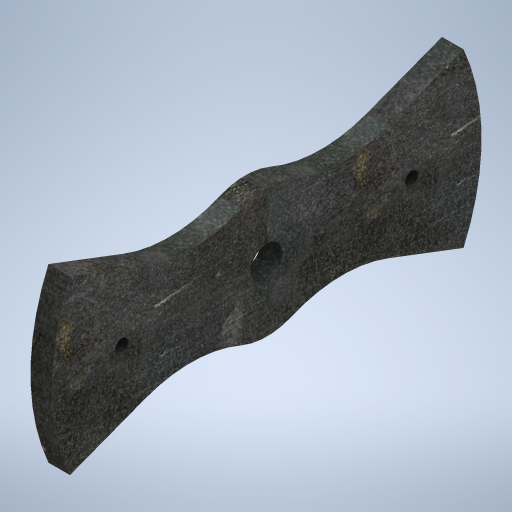
# Autodesk Inventor part: Test weapon
Saved by Autodesk Inventor 2023 (Build 270158000, 158)
## iProperties
Created: 2023-01-06
Part Number: Test weapon
Material: Steel
Document SubType Name: Modeling
Designer: justi
Density: 7.85 g/cm^3
Appearance: Plate
Mass: 1776.63 g
Surface Area: 458.545 cm^2
Volume: 226.322 cm^3
Author: justi
Autodesk Inventor part; units mm, degrees
ref_plane "YZ Plane" through (0, 0, 0) normal (1, 0, 0) x (0, 1, 0)
ref_plane "XZ Plane" through (0, 0, 0) normal (0, 1, 0) x (-1, 0, 0)
ref_plane "XY Plane" through (0, 0, 0) normal (0, 0, 1) x (1, 0, 0)
sketch "Sketch1" plane through (0, 0, 0) normal (1, 0, 0) x (0, 1, 0)
  circle A0 centre (0, 0) radius 38.1
  circle A1 centre (0, 0) radius 9.525
  circle A2 centre (0, 0) radius 127
  line L0 (-19.05, 127) -> (19.05, 127)
  line L1 (19.05, 127) -> (19.05, -127)
  line L2 (19.05, -127) -> (-19.05, -127)
  line L3 (-19.05, -127) -> (-19.05, 127)
  line L4 (-19.05, 127) -> (19.05, -127) construction
  line L5 (19.05, 127) -> (-19.05, -127) construction
  line L6 (-50.8, 127) -> (50.8, 127)
  line L7 (50.8, 127) -> (50.8, -127)
  line L8 (50.8, -127) -> (-50.8, -127)
  line L9 (-50.8, -127) -> (-50.8, 127)
  line L10 (-50.8, 127) -> (50.8, -127) construction
  line L11 (50.8, 127) -> (-50.8, -127) construction
  line L12 (19.05, 32.9956) -> (50.8, 116.3974)
  line L13 (-19.05, 32.9956) -> (-50.8, 116.3974)
  line L14 (19.05, -32.9956) -> (50.8, -116.3974)
  line L15 (-19.05, -32.9956) -> (-50.8, -116.3974)
  dimension "d0" = 76.2
  dimension "d1" = 19.05
  dimension "d2" = 254
  dimension "d3" = 38.1
  dimension "d4" = 254
  dimension "d5" = 101.6
  dimension "d6" = 254
  constraints: 32 end point, 8 point on circle, 8 point on line, 4 midpoint, 4 parallel, 3 centre point, 3 coincident, 2 horizontal, 2 perpendicular
  measures "d0" diameter of A0
  measures "d1" diameter of A1
  measures "d2" diameter of A2
  measures "d3" distance of L1.end L2.end
  measures "d4" distance of L0.end L1.end
  measures "d5" distance of L7.end L8.end
  measures "d6" distance of L6.end L7.end
extrude "Extrusion1" add sketch "Sketch1" along normal blind 12.7 contours A0 L1 | L1 A0 L3 | A0 L3 A2 L1 | L1 A2 L12 | L1 A2 L3 A0 | L14 A2 L1 | L3 A0 | L13 A2 L3 | L3 A2 L15
fillet "Fillet1" radius 76.2 4 edges at (6.35, 19.05, 32.9956) (6.35, -19.05, 32.9956) (6.35, -19.05, -32.9956) (6.35, 19.05, -32.9956)
sketch "Sketch3" plane through (12.7, 0, 0) normal (1, 0, 0) x (0, 0, -1)
  circle A0 centre (-85.725, 0) radius 3.9688
  circle A1 centre (-114.3, 0) radius 4.7625 projected
  circle A2 centre (85.725, 0) radius 3.9687
  circle A3 centre (114.3, 0) radius 4.7625 projected
  point P0 (0, 0)
  dimension "d47" = 7.9375
  dimension "d48" = 28.575
  dimension "d49" = 7.9375
  dimension "d50" = 28.575
  constraints: 2 centre point
  measures "d47" diameter of A0
  measures "d48" distance of A1.centre A0.centre
  measures "d49" diameter of A2
  measures "d50" distance of A3.centre A2.centre
extrude "Extrusion3" cut sketch "Sketch3" against normal blind 12.7 contours A0 | A2
body "Solid1"
